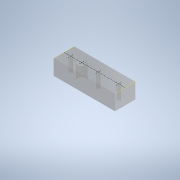
# Autodesk Inventor part: BOt
Saved by Autodesk Inventor 2020 (Build 240168000, 168)
## iProperties
Created: 2019-02-01
Part Number: BOt
Material: 일반
Document SubType Name: Modeling
Designer: Jeong Ji Hoon
Density: 1 g/cm^3
Appearance: 연회색 반사
Author: Jeong Ji Hoon
Autodesk Inventor part; units mm, degrees
ref_plane "YZ Plane" through (0, 0, 0) normal (1, 0, 0) x (0, 1, 0)
ref_plane "XZ Plane" through (0, 0, 0) normal (0, 1, 0) x (-1, 0, 0)
ref_plane "XY Plane" through (0, 0, 0) normal (0, 0, 1) x (1, 0, 0)
sketch "스케치1" plane through (0, 0, 0) normal (0, 1, 0) x (-1, 0, 0)
  line L0 (0, 0) -> (12, 0)
  line L1 (12, 0) -> (12, -4)
  line L2 (12, -4) -> (0, -4)
  line L3 (0, -4) -> (0, 0)
  dimension "d0" = 12
  dimension "d1" = 4
  constraints: 8 end point, 2 parallel, 1 horizontal, 1 perpendicular
  measures "d0" distance of L1.end L2.end
  measures "d1" distance of L0.end L1.end
extrude "돌출1" add sketch "스케치1" along normal blind 3
sketch "스케치2" plane through (0, 3, 0) normal (0, 1, 0) x (1, 0, 0)
  line L0 (0, 0) -> (0, 4) construction
  line L1 (0, 2) -> (-12, 2) construction
  line L2 (-12, 4) -> (-12, 0) construction
  point P0 (-1.3, 2)
  point P1 (-5.3, 2)
  point P2 (-8.5, 2)
  point P3 (-10.7, 2)
  dimension "d59" = 1.3
  dimension "d60" = 2.2
  dimension "d61" = 3.2
  dimension "d62" = 1.3
  constraints: 4 point on line, 2 end point, 2 midpoint
  measures "d59" distance from line of L2 point (-10.7, 2)
  measures "d60" distance of point (-10.7, 2) point (-8.5, 2)
  measures "d61" distance of point (-5.3, 2) point (-8.5, 2)
  measures "d62" distance from line of L0 point (-1.3, 2)
hole "구멍1" at (-10.7, 3, -2) at (-1.3, 3, -2) direction (0, -1, 0) diameter 0.65 end through all
hole "구멍2" at (-8.5, 3, -2) direction (0, -1, 0) diameter 1.6 end through all
hole "구멍3" at (-5.3, 3, -2) direction (0, -1, 0) diameter 0.63 end through all
equation "\"G23_F\" = 0.65"
equation "\"G23_M\" = 0.67"
equation "\"Screw_F\" = 1.3"
equation "\"Screw_M\" = 1.6"
